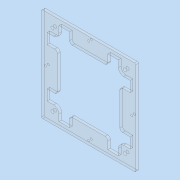
# Autodesk Inventor part: WaagePlexiOben1
Saved by Autodesk Inventor 2022 (Build 260153000, 153)
## iProperties
Created: 2021-12-03
Part Number: WaagePlexiOben1
Material: PET Plastic
Document SubType Name: Modeling
Designer: domin
Density: 1.541 g/cm^3
Appearance: Polycarbonate - Clear
Mass: 110.779 g
Surface Area: 366.745 cm^2
Volume: 71.8875 cm^3
Author: domin
Autodesk Inventor part; units mm, degrees
ref_plane "YZ Plane" through (0, 0, 0) normal (1, 0, 0) x (0, 1, 0)
ref_plane "XZ Plane" through (0, 0, 0) normal (0, 1, 0) x (-1, 0, 0)
ref_plane "XY Plane" through (0, 0, 0) normal (0, 0, 1) x (1, 0, 0)
sketch "Sketch1" plane through (0, 0, 0) normal (0, 0, 1) x (1, 0, 0)
  line L0 (-89, 89) -> (89, 89)
  line L1 (89, 89) -> (89, -89)
  line L2 (89, -89) -> (-89, -89)
  line L3 (-89, -89) -> (-89, 89)
  line L4 (-56.125, 56.125) -> (-78.5, 56.125)
  line L5 (-78.5, -56.125) -> (-56.125, -56.125)
  line L6 (56.125, 56.125) -> (56.125, 78.5)
  line L7 (-56.125, 78.5) -> (-56.125, 56.125)
  line L8 (56.125, 56.125) -> (78.5, 56.125)
  line L9 (78.5, -56.125) -> (56.125, -56.125)
  line L10 (56.125, -56.125) -> (56.125, -78.5)
  line L11 (-56.125, -78.5) -> (-56.125, -56.125)
  line L12 (-78.5, 36.125) -> (-59, 36.125)
  line L13 (-59, 36.125) -> (-59, -36.125)
  line L14 (-59, -36.125) -> (-78.5, -36.125)
  line L15 (-78.5, 56.125) -> (-78.5, 36.125)
  line L16 (-78.5, -36.125) -> (-78.5, -56.125)
  line L17 (78.5, 36.125) -> (59, 36.125)
  line L18 (59, 36.125) -> (59, -36.125)
  line L19 (59, -36.125) -> (78.5, -36.125)
  line L20 (78.5, 56.125) -> (78.5, 36.125)
  line L21 (78.5, -36.125) -> (78.5, -56.125)
  line L22 (36.125, 78.5) -> (36.125, 59)
  line L23 (36.125, 59) -> (-36.125, 59)
  line L24 (-36.125, 59) -> (-36.125, 78.5)
  line L25 (36.125, -78.5) -> (36.125, -59)
  line L26 (36.125, -59) -> (-36.125, -59)
  line L27 (-36.125, -59) -> (-36.125, -78.5)
  line L28 (56.125, 78.5) -> (36.125, 78.5)
  line L29 (-36.125, 78.5) -> (-56.125, 78.5)
  line L30 (56.125, -78.5) -> (36.125, -78.5)
  line L31 (-36.125, -78.5) -> (-56.125, -78.5)
  point P0 (0, 0)
  point P1 (-78.5, 0)
  dimension "d4" = 112.25
  dimension "d5" = 112.25
  dimension "d29" = 0
  dimension "d30" = 0
  dimension "d33" = 178
  dimension "d34" = 89
  dimension "d35" = 89
  dimension "d41" = 20
  dimension "d42" = 20
  dimension "d43" = 30
  dimension "d46" = 20
  dimension "d47" = 20
  dimension "d48" = 30
  dimension "d49" = 157
  dimension "d50" = 78.5
  dimension "d51" = 30
  dimension "d52" = 30
  dimension "d53" = 20
  dimension "d54" = 157
  dimension "d55" = 78.5
  dimension "d56" = 20
  constraints: 64 end point, 10 parallel, 8 coincident, 7 horizontal, 7 horizontal alignment, 7 perpendicular, 7 vertical alignment, 6 equal length, 2 point on line, 16 other
  measures "d29" vertical extent of L4
  measures "d30" distance from line of point (-56.125, 56.125) L7
  measures "d33" distance between parallel lines of L1 L3
  measures "d34" distance from line of point (0, 0) L0
  measures "d35" distance from line of point (0, 0) L3
  measures "d41" distance between parallel lines of L12 L4
  measures "d42" distance between parallel lines of L5 L14
  measures "d43" distance between parallel lines of L3 L13
  measures "d46" distance between parallel lines of L17 L8
  measures "d47" distance between parallel lines of L9 L19
  measures "d48" distance between parallel lines of L1 L18
  measures "d49" distance between parallel lines of L20 L15
  measures "d50" distance from line of point (0, 0) L15
  measures "d51" distance between parallel lines of L23 L0
  measures "d52" distance between parallel lines of L2 L26
  measures "d53" distance between parallel lines of L6 L22
  measures "d54" distance between parallel lines of L31 L29
  measures "d55" distance from line of point (0, 0) L29
  measures "d56" distance between parallel lines of L24 L7
extrude "Extrusion1" add sketch "Sketch1" along normal blind 5
sketch "Sketch2" plane through (0, 0, 5) normal (0, 0, 1) x (1, 0, 0)
  circle A0 centre (-81.5, 0) radius 2
  circle A1 centre (81.5, 0) radius 2
  line L0 (-78.5, 36.125) -> (-78.5, 56.125) projected
  line L1 (78.5, 56.125) -> (78.5, 36.125) projected
  circle A2 centre (0, 81.5) radius 2
  circle A3 centre (0, -81.5) radius 2
  line L2 (36.125, 78.5) -> (56.125, 78.5) projected
  line L3 (56.125, -78.5) -> (36.125, -78.5) projected
  line L4 (-89, 89) -> (-89, -89) projected
  line L5 (89, 89) -> (-89, 89) projected
  line L6 (89, -89) -> (89, 89) projected
  line L7 (-89, -89) -> (89, -89) projected
  point P0 (0, 0)
  point P1 (-78.5, -56.125)
  point P2 (78.5, -56.125)
  point P3 (-56.125, 78.5)
  point P4 (-56.125, -78.5)
  dimension "d18" = 4
  dimension "d37" = 7.5
  dimension "d38" = 7.5
  dimension "d39" = 7.5
  dimension "d40" = 7.5
  constraints: 4 centre point, 3 equal radius, 2 horizontal alignment, 2 vertical alignment
  measures "d18" diameter of A0
  measures "d37" distance from line of A0.centre L4
  measures "d38" distance from line of L5 A2.centre
  measures "d39" distance from line of L6 A1.centre
  measures "d40" distance from line of L7 A3.centre
hole "Hole1" at (-81.5, 0, 5) at (0, 81.5, 5) at (81.5, 0, 5) at (0, -81.5, 5) direction (0, 0, -1) diameter 4 end through all
fillet "Fillet1" radius 2 4 edges at (-89, -89, 2.5) (-89, 89, 2.5) (89, -89, 2.5) (89, 89, 2.5)
sketch "Sketch3" plane through (0, 0, 5) normal (0, 0, 1) x (1, 0, 0)
  line L0 (68.475, -68.475) -> (-68.475, -68.475)
  line L1 (-68.475, -68.475) -> (-68.475, 68.475)
  line L2 (-68.475, 68.475) -> (68.475, 68.475)
  line L3 (68.475, 68.475) -> (68.475, -68.475)
  line L4 (68.475, -68.475) -> (-68.475, 68.475) construction
  line L5 (-68.475, -68.475) -> (68.475, 68.475) construction
  circle A0 centre (-68.475, 68.475) radius 4.875
  point P0 (0, 0)
  dimension "d31" = 136.95
  dimension "d32" = 9.75
  constraints: 12 end point, 2 midpoint, 2 parallel, 2 perpendicular, 1 centre point, 1 coincident, 1 horizontal
  measures "d31" distance of L1.end L2.end
  measures "d32" diameter of A0
fillet "Fillet2" radius 10 4 edges at (-56.125, 56.125, 2.5) (56.125, 56.125, 2.5) (56.125, -56.125, 2.5) (-56.125, -56.125, 2.5)
fillet "Fillet3" radius 5 8 edges at (-59, 36.125, 2.5) (-59, -36.125, 2.5) (-36.125, -59, 2.5) (36.125, -59, 2.5) (59, -36.125, 2.5) (59, 36.125, 2.5) (36.125, 59, 2.5) (-36.125, 59, 2.5)
hole "Hole2" at (-68.475, 68.475, 5) at (68.475, 68.475, 5) at (68.475, -68.475, 5) at (-68.475, -68.475, 5) direction (0, 0, -1) diameter 6 end through all
equation "\"d34\" = 0.5 * d33"
equation "\"d35\" = 0.5 * d33"
equation "\"d50\" = 0.5 * d49"
equation "\"d55\" = 0.5 * d54"
equation "\"d38\" = d37"
equation "\"d39\" = d37"
equation "\"d40\" = d37"
equation "\"d21\" = d18"
equation "\"d6\" = 0.5 * d3"
equation "\"d7\" = 0.5 * d2"
equation "\"d3\" = 157"
equation "\"d2\" = 157"
body "Solid1"
